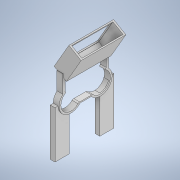
# Autodesk Inventor part: ultrasonic_fastening
Saved by Autodesk Inventor 2022 (Build 260153000, 153)
## iProperties
Created: 2022-02-09
Part Number: ultrasonic_fastening
Material: Generic
Document SubType Name: Modeling
Designer: Iñigo
Density: 1 g/cm^3
Appearance: Default
Author: Iñigo
Autodesk Inventor part; units mm, degrees
ref_plane "YZ Plane" through (0, 0, 0) normal (1, 0, 0) x (0, 1, 0)
ref_plane "XZ Plane" through (0, 0, 0) normal (0, 1, 0) x (-1, 0, 0)
sketch "Sketch3" plane through (0, 0, 0) normal (1, 0, 0) x (0, 1, 0)
  arc A0 (7.6059, 16.7425) -> (-5.7973, 6.5139) centre (0.2447, 12.4925) ccw
  arc A1 (8.905, 17.4925) -> (-6.7785, 5.374) centre (0.2447, 12.4925) ccw
  line L0 (8.7447, -0.0075) -> (4.3518, -0.0075)
  line L1 (0.2447, 12.4925) -> (0.2447, 2.4925) construction
  line L2 (0.2447, 12.4925) -> (0.2447, 2.4925) construction
  line L3 (8.905, 17.4925) -> (7.6059, 16.7425)
  arc A2 (-6.7785, -5.3889) -> (8.905, -17.5075) centre (0.2447, -12.5075) ccw
  arc A3 (-5.7973, -6.5288) -> (7.6059, -16.7575) centre (0.2447, -12.5075) ccw
  line L4 (8.905, -17.5075) -> (7.6059, -16.7575)
  line L5 (-5.219, 5.1072) -> (-5.219, -5.1221)
  line L6 (-6.1832, 3.9502) -> (-6.1832, -3.9652)
  arc A4 (-5.219, 5.1072) -> (-5.7973, 6.5139) centre (-7.219, 5.1072) ccw
  arc A5 (-5.7973, -6.5288) -> (-5.219, -5.1221) centre (-7.219, -5.1221) ccw
  arc A6 (-6.1832, 3.9502) -> (-6.7785, 5.374) centre (-8.1832, 3.9502) ccw
  arc A7 (-6.7785, -5.3889) -> (-6.1832, -3.9652) centre (-8.1832, -3.9652) ccw
  point P0 (0, 0)
  point P1 (0.2447, -0.2026)
  point P2 (-6.1832, 4.8321)
  point P3 (-6.1832, -4.847)
  point P4 (-5.219, -5.9961)
  point P5 (-6.1832, -4.847)
  dimension "d18" = 20
  dimension "d19" = 12.5
  dimension "d20" = 2
  dimension "d21" = 2
  constraints: 18 point on circle, 14 end point, 8 centre point, 8 tangent, 5 symmetric about line, 3 point on line, 2 coincident, 2 equal radius, 2 other
  measures "d18" diameter of A1
  measures "d19" distance from line of A0.centre L0
  measures "d20" radius of A4
  measures "d21" radius of A6
extrude "Extrusion3" add sketch "Sketch3" along normal blind 5
ref_plane "Work Plane3" through (0, 0, 22) normal (0, 0, 1) x (1, 0, 0)
sketch "Sketch4" plane through (0, 0, 22) normal (0, 0, 1) x (1, 0, 0)
  line L0 (0, 0) -> (4, 0)
  line L1 (4, 0) -> (4, -40)
  line L2 (4, -40) -> (0, -40)
  line L3 (0, -40) -> (0, 0)
  dimension "d26" = 40
  constraints: 8 end point, 2 parallel, 1 horizontal, 1 perpendicular
  measures "d26" distance of L0.end L1.end
extrude "Extrusion4" add sketch "Sketch4" along normal blind 3
sketch "Sketch5" plane through (0, 0, 22) normal (0, 0, -1) x (-1, 0, 0)
  line L0 (0, -8.2553) -> (0, 7.6059) projected
  line L1 (-4, -40) -> (0, -40)
  line L2 (0, -40) -> (0, -2.5366)
  line L3 (0, -2.5366) -> (-4, -2.5366)
  line L4 (-4, -2.5366) -> (-4, -40)
  point P0 (0, 0)
  point P1 (0, -5.7973)
  constraints: 8 end point, 2 parallel, 1 horizontal, 1 perpendicular, 1 point on line
extrude "Extrusion5" add sketch "Sketch5" along normal blind 9
sketch "Sketch6" plane through (4, -8.2401, 13) normal (1, 0, 0) x (0, 0, -1)
  line L0 (-7.5246, 5.7036) -> (0, 5.7036) projected
  line L1 (0, 5.7036) -> (0, 0) projected
  arc A0 (0, 0) -> (6.4861, 2.4428) centre (0.5075, 8.4848) ccw projected
  arc A1 (-7.5246, 5.7036) -> (0, 0) centre (0.5075, 8.4848) ccw
  line L2 (-7.5246, 5.7036) -> (0, 5.7036)
  line L3 (0, 0) -> (0, 5.7036)
  point P0 (13, 8.2401)
  constraints: 4 end point, 2 collinear, 2 point on circle, 1 centre point
extrude "Extrusion6" cut sketch "Sketch6" against normal blind 4
mirror "Mirror1" about plane through (0, 0, 0) normal (0, 0, 1) of "Extrusion4", "Extrusion5", "Extrusion6"
sketch "Sketch7" plane through (0, 0, 0) normal (1, 0, 0) x (0, 1, 0)
  line L0 (7.4997, 17.4925) -> (22.4997, 17.4925)
  line L1 (22.4997, 17.4925) -> (22.4997, 19.3358)
  line L2 (22.4997, 19.3358) -> (7.4997, 19.3358)
  line L3 (7.4997, 19.3358) -> (7.4997, 17.4925)
  line L4 (7.4997, -17.4925) -> (22.4997, -17.4925)
  line L5 (22.4997, -17.4925) -> (22.4997, -19.3358)
  line L6 (22.4997, -19.3358) -> (7.4997, -19.3358)
  line L7 (7.4997, -19.3358) -> (7.4997, -17.4925)
  point P0 (0, 0)
  dimension "d34" = 15
  constraints: 16 end point, 2 parallel, 1 horizontal, 1 perpendicular
  measures "d34" distance of L2.end L1.end
extrude "Extrusion7" add sketch "Sketch7" along normal blind 5
sketch "Sketch8" plane through (0, 8.905, 17.4925) normal (0, 0, -1) x (-1, 0, 0)
  line L0 (0, 13.5948) -> (-5, 13.5948) projected
  line L1 (2.7357, 15.1738) -> (-9.7741, 36.8188)
  line L2 (2.7357, 15.1738) -> (27.7357, 15.1738) construction
  line L3 (-9.7741, 36.8188) -> (-20.1665, 30.8189)
  line L4 (-20.1665, 30.8189) -> (-7.6667, 9.1681)
  line L5 (0, 0) -> (0, 13.5948) projected
  line L6 (-7.6667, 9.1681) -> (2.7357, 15.1738)
  point P0 (0, -8.905)
  dimension "d37" = 25.197
  dimension "d39" = 12
  dimension "d40" = 25
  constraints: 10 end point, 2 perpendicular, 1 equal length, 1 horizontal
  measures "d37" distance of L0.start L1.end
  measures "d39" distance of L1.end L3.end
  measures "d40" distance of L3.end L4.end
extrude "Extrusion8" add sketch "Sketch8" along normal blind 36.5
sketch "Sketch9" plane through (0, 8.905, 17.4925) normal (0, 0, 1) x (1, 0, 0)
  line L0 (0, 0) -> (0, 13.5948)
  line L1 (0, 13.5948) -> (5, 13.5948)
  line L2 (-2.7357, 15.1738) -> (9.7741, 36.8188)
  line L3 (9.7741, 36.8188) -> (20.1665, 30.8189)
  line L4 (20.1665, 30.8189) -> (7.6667, 9.1681)
  line L5 (7.6667, 9.1681) -> (-2.7357, 15.1738)
  point P0 (0, -8.905)
  constraints: 12 end point
extrude "Extrusion9" add sketch "Sketch9" along normal blind 1.5
sketch "Sketch10" plane through (20.1665, 39.7238, 18.9925) normal (0.4999921, 0.86603, 0) x (0.86603, -0.4999921, 0)
  line L0 (-12, 0) -> (-12, 38) projected
  line L1 (-12, 38) -> (0, 38) projected
  line L2 (-12, 0) -> (0, 0)
  line L3 (0, 0) -> (0, 38)
  line L4 (0, 38) -> (-12, 38)
  line L5 (-12, 38) -> (-12, 0)
  line L6 (-11, 1.5) -> (-1, 1.5)
  line L7 (-1, 1.5) -> (-1, 36.5)
  line L8 (-1, 36.5) -> (-11, 36.5)
  line L9 (-11, 36.5) -> (-11, 1.5)
  point P0 (2.3968, 18.9925)
  dimension "d51" = 10
  dimension "d52" = 35
  constraints: 16 end point, 4 parallel, 2 horizontal, 2 perpendicular
  measures "d51" distance of L8.end L7.end
  measures "d52" distance of L7.end L6.end
extrude "Extrusion10" cut sketch "Sketch10" against normal blind 24 contours L9 L8 L7 L6
sketch "Sketch11" plane through (9.7741, 45.7238, -19.0075) normal (-0.8657981, 0.5003936, 0) x (0, 0, 1)
  line L0 (0, 0.0056) -> (0, -24.9944) projected
  line L1 (38.3433, -22.4963) -> (38.3433, -35.4514) projected
  line L2 (0, 0.0056) -> (38.3433, 0.0056)
  line L3 (38.3433, 0.0056) -> (38.3433, -25.0729)
  line L4 (38.3433, -25.0729) -> (0, -25.0729)
  line L5 (0, -25.0729) -> (0, 0.0056)
  line L6 (1.6716, -1.5337) -> (36.6716, -1.5337)
  line L7 (36.6716, -1.5337) -> (36.6716, -23.5337)
  line L8 (36.6716, -23.5337) -> (1.6716, -23.5337)
  line L9 (1.6716, -23.5337) -> (1.6716, -1.5337)
  line L10 (1.6716, -1.5337) -> (36.6716, -23.5337) construction
  line L11 (36.6716, -1.5337) -> (1.6716, -23.5337) construction
  point P0 (19.0075, -44.4784)
  point P1 (19.1716, -12.5337)
  dimension "d55" = 35
  dimension "d56" = 22
  constraints: 20 end point, 4 parallel, 2 horizontal, 2 midpoint, 2 perpendicular, 1 point on line
  measures "d55" distance of L7.end L8.end
  measures "d56" distance of L6.end L7.end
extrude "Extrusion11" cut sketch "Sketch11" against normal blind 3.75 contours L6 L7 L8 L9
body "Solid2"
